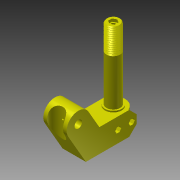
# Autodesk Inventor part: hub bottom
Saved by Autodesk Inventor 2013 (Build 170138000, 138)
## iProperties
Created: 2013-07-14
Part Number: hub bottom
Material: Generic
Document SubType Name: Modeling
Designer: employee
Density: 1 g/cm^3
Author: employee
Autodesk Inventor part; units mm, degrees
ref_plane "YZ Plane" through (0, 0, 0) normal (1, 0, 0) x (0, 1, 0)
ref_plane "XZ Plane" through (0, 0, 0) normal (0, 1, 0) x (-1, 0, 0)
ref_plane "XY Plane" through (0, 0, 0) normal (0, 0, 1) x (1, 0, 0)
sketch "Sketch1" plane through (0, 0, 0) normal (1, 0, 0) x (0, 1, 0)
  circle A0 centre (-50, 14) radius 4.05
  arc A1 (-39.174682, 20.25) -> (-60.825318, 7.75) centre (-50, 14) ccw
  line L0 (0, 0) -> (0, -25)
  line L1 (0, -25) -> (-41.917096, -25)
  line L2 (-41.917096, -25) -> (-60.825318, 7.75)
  line L3 (0, 0) -> (-27.48334, 0)
  line L4 (-27.48334, 0) -> (-39.174682, 20.25)
  dimension "d0" = 8.1
  dimension "d2" = 50
  dimension "d3" = 14
  dimension "d4" = 25
  dimension "d6" = 25
  dimension "d40" = 120
  constraints: 10 end point, 2 centre point, 2 parallel, 2 point on circle, 2 tangent, 1 coincident, 1 perpendicular, 1 vertical
  measures "d0" diameter of A0
  measures "d2" horizontal distance of L0.start A0.centre
  measures "d3" vertical distance of A0.centre L0.start
  measures "d4" diameter of A1
  measures "d6" distance of L0.start L0.end
  measures "d40" angle of L2 L1
extrude "Extrusion1" add sketch "Sketch1" along normal mid plane 25
sketch "Sketch2" plane through (-12.5, -27.48334, 0) normal (0, 0, 1) x (1, 0, 0)
  circle A0 centre (12.5, 27.48334) radius 12.5
  constraints: 1 centre point, 1 coincident
extrude "Extrusion2" add sketch "Sketch2" against normal up to surface (25 mm away)
sketch "Sketch13" plane through (12.5, 0, 0) normal (1, 0, 0) x (0, 0, -1)
  line L0 (0, 0) -> (0, -27.48334)
  line L1 (25, 0) -> (0, 0)
  line L2 (25, 0) -> (25, 0)
  line L3 (0, 0) -> (25, 0)
  line L4 (0, 0) -> (0, 0)
  line L5 (0, 12.5) -> (25, 12.5)
  line L6 (0, 0) -> (0, 12.5)
  line L7 (25, 12.5) -> (25, 0)
  line L8 (0, 4.5) -> (8, 12.5)
  line L9 (17, 12.5) -> (25, 4.5)
  line L10 (0, 0) -> (0, 4.5)
  line L11 (0, 0) -> (25, 0)
  line L12 (25, 0) -> (25, 4.5)
  line L13 (17, 12.5) -> (8, 12.5)
  dimension "d60" = 45
  dimension "d61" = 9
  constraints: 12 end point, 4 perpendicular, 4 point on line, 1 collinear, 1 parallel
  measures "d60" angle of L5 L8
  measures "d61" distance of L9.start L8.end
extrude "Extrusion13" add sketch "Sketch13" against normal up to surface (25 mm away) contours L1 L6 L8 L5 L9 L7
sketch "Sketch12" plane through (12.5, -41.917096, -25) normal (0, 0, -1) x (-1, 0, 0)
  arc A0 (25, 41.917096) -> (0, 41.917096) centre (12.5, 41.917096) ccw
  circle A1 centre (12.5, 41.917096) radius 8.1
  dimension "d56" = 16.2
  constraints: 1 centre point, 1 coincident
  measures "d56" diameter of A1
extrude "Extrusion12" cut sketch "Sketch12" against normal blind 19
sketch "Sketch14" plane through (-12.5, 0, 0) normal (-1, 0, 0) x (0, 0, 1)
  line L0 (-8, 12.5) -> (-17, 12.5) projected
  line L1 (-6, -8.1) -> (-6, 8.1) projected
  line L2 (-25, -8.1) -> (-25, 8.1) projected
  line L3 (-25, 8.1) -> (-6, 8.1) projected
  line L4 (-25, -8.1) -> (-6, -8.1) projected
  line L5 (-12.5, 7.25) -> (-12.5, -7.25)
  circle A0 centre (-12.5, 7.25) radius 1.55
  circle A1 centre (-12.5, -7.25) radius 1.55
  point P0 (0, 0)
  point P1 (-6, -0.010608)
  point P2 (-6, 0)
  point P3 (-12.5, 0)
  point P4 (-12.5, 12.5)
  dimension "d65" = 3.1
  dimension "d67" = 14.5
  constraints: 3 midpoint, 2 centre point, 2 coincident, 2 end point, 2 vertical alignment, 1 equal radius, 1 horizontal alignment, 1 perpendicular
  measures "d65" diameter of A1
  measures "d67" distance of L5.start L5.end
extrude "Extrusion14" cut sketch "Sketch14" against normal through all contours A1 L4 | L4 A1 | A0 L3 | L3 A0
sketch "Sketch15" plane through (-12.5, 0, 0) normal (-1, 0, 0) x (0, 0, 1)
  circle A0 centre (-12.5, -7.25) radius 1.55 projected
  circle A1 centre (-12.5, 7.25) radius 1.55 projected
  circle A2 centre (-12.5, 7.25) radius 3.25
  circle A3 centre (-12.5, -7.25) radius 3.25
  point P0 (0, 0)
  dimension "d70" = 6.5
  constraints: 2 centre point, 2 coincident, 1 equal radius
  measures "d70" diameter of A3
extrude "Extrusion15" cut sketch "Sketch15" against normal blind 4
sketch "Sketch16" plane through (12.5, 0, 0) normal (1, 0, 0) x (0, 0, -1)
  circle A0 centre (12.5, -7.25) radius 1.55
  circle A1 centre (12.5, 7.25) radius 1.55
  line L0 (12.5, -10.483162) -> (9.7, -8.866581)
  line L1 (9.7, -8.866581) -> (9.7, -5.633419)
  line L2 (9.7, -5.633419) -> (12.5, -4.016838)
  line L3 (12.5, -4.016838) -> (15.3, -5.633419)
  line L4 (15.3, -5.633419) -> (15.3, -8.866581)
  line L5 (15.3, -8.866581) -> (12.5, -10.483162)
  line L6 (12.5, 4.016838) -> (9.7, 5.633419)
  line L7 (9.7, 5.633419) -> (9.7, 8.866581)
  line L8 (9.7, 8.866581) -> (12.5, 10.483162)
  line L9 (12.5, 10.483162) -> (15.3, 8.866581)
  line L10 (15.3, 8.866581) -> (15.3, 5.633419)
  line L11 (15.3, 5.633419) -> (12.5, 4.016838)
  point P0 (0, 0)
  dimension "d74" = 5.6
  constraints: 24 end point, 2 coincident, 2 vertical, 1 collinear, 26 other
  measures "d74" distance between parallel lines of L4 L1
extrude "Extrusion16" cut sketch "Sketch16" against normal blind 4
sketch "Sketch17" plane through (-12.5, -27.48334, 0) normal (0, 0, 1) x (1, 0, 0)
  arc A0 (24.161904, 31.98334) -> (0.838096, 31.98334) centre (12.5, 27.48334) ccw
  circle A1 centre (12.5, 27.48334) radius 9
  point P0 (23.286001, 33.800949)
  point P1 (1.713999, 33.800949)
  dimension "d77" = 18
  constraints: 1 centre point, 1 coincident
  measures "d77" diameter of A1
extrude "Extrusion17" add sketch "Sketch17" along normal blind 1.5
sketch "Sketch18" plane through (0, 0, 1.5) normal (0, 0, 1) x (1, 0, 0)
  circle A0 centre (0, 0) radius 9 projected
  circle A1 centre (0, 0) radius 7.35
  dimension "d82" = 14.7
  constraints: 1 centre point, 1 coincident
  measures "d82" diameter of A1
extrude "Extrusion18" add sketch "Sketch18" along normal blind 76.5 contours A1
sketch "Sketch19" plane through (0, 0, 0) normal (1, 0, 0) x (0, 1, 0)
  line L0 (12.5, -17) -> (12.5, -25)
  line L1 (12.5, -25) -> (8.1, -25)
  line L2 (8.1, -25) -> (8.1, -13.796148)
  arc A0 (8.1, -13.796148) -> (8.1, -11.203852) centre (7.25, -12.5) ccw
  line L3 (8.1, -11.203852) -> (8.1, -6)
  line L4 (8.1, -6) -> (-8.1, -6)
  line L5 (-8.1, -6) -> (-8.1, -11.203852)
  arc A1 (-8.1, -11.203852) -> (-8.1, -13.796148) centre (-7.25, -12.5) ccw
  line L6 (-8.1, -13.796148) -> (-8.1, -25)
  line L7 (-8.1, -25) -> (-41.917096, -25)
  line L8 (-41.917096, -25) -> (-60.825318, 7.75)
  arc A2 (-39.174682, 20.25) -> (-60.825318, 7.75) centre (-50, 14) ccw
  line L9 (-39.174682, 20.25) -> (-27.48334, 0)
  line L10 (-27.48334, 0) -> (-9, 0)
  line L11 (-9, 0) -> (-9, 1.5)
  line L12 (-9, 1.5) -> (-7.35, 1.5)
  line L13 (-7.35, 1.5) -> (-7.35, 78)
  line L14 (-7.35, 78) -> (7.35, 78)
  line L15 (7.35, 78) -> (7.35, 1.5)
  line L16 (7.35, 1.5) -> (9, 1.5)
  line L17 (9, 1.5) -> (9, 0)
  line L18 (9, 0) -> (12.5, 0)
  line L19 (12.5, 0) -> (12.5, -8)
  line L20 (12.5, -8) -> (12.5, -17)
  circle A3 centre (-50, 14) radius 4.05
  line L21 (7.35, 78) -> (7.35, 80)
  line L22 (7.35, 80) -> (6.35, 79)
  line L23 (6.35, 79) -> (7.35, 78)
  line L24 (0, 78) -> (0, 72.188815)
  point P0 (0, 0)
  dimension "d87" = 2
  constraints: 8 end point, 2 parallel, 2 perpendicular, 1 midpoint
  measures "d87" distance of L14.end L21.end
coil "Coil1" sketch "Sketch19" operation cut axis through (0, 0, 78) along (0, 0, -1) pitch 2.001 turns 30 hand right contours L23 L22 L21
sketch "Sketch20" plane through (0, 0, 1.5) normal (0, 0, 1) x (1, 0, 0)
  circle A0 centre (0, 0) radius 7.35 projected
extrude "Extrusion19" add sketch "Sketch20" along normal blind 49.5
sketch "Sketch21" plane through (0, 0, 51) normal (0, 0, 1) x (1, 0, 0)
  arc A0 (0.334532, -7.342383) -> (0.311475, -7.343397) centre (0, 0) ccw
  circle A1 centre (0, 0) radius 7.35
  constraints: 1 centre point, 1 coincident, 1 concentric
extrude "Extrusion20" add sketch "Sketch21" along normal blind 5 draft -45
sketch "Sketch22" plane through (0, 0, 78) normal (0, 0, 1) x (1, 0, 0)
  arc A0 (0, 7.35) -> (-0.023079, 7.349964) centre (0, 0) ccw
  circle A1 centre (0, 0) radius 6.45
  circle A2 centre (0, 0) radius 20
  dimension "d100" = 40
  constraints: 2 centre point, 2 coincident
  measures "d100" diameter of A2
extrude "Extrusion21" cut sketch "Sketch22" against normal blind 5 draft -45
sketch "Sketch23" plane through (0, 0, 78) normal (0, 0, 1) x (-0.9999988, -0.00157, 0)
  circle A0 centre (0, 0) radius 6.45 projected
  circle A1 centre (0, 0) radius 2.5
  point P0 (0.010127, -6.449992)
  dimension "d104" = 5
  constraints: 1 centre point, 1 coincident, 1 other
  measures "d104" diameter of A1
extrude "Extrusion22" cut sketch "Sketch23" against normal through all contours A1
sketch "Sketch24" plane through (0, 0, -6) normal (0, 0, -1) x (-1, 0, 0)
  circle A0 centre (0, 0) radius 2.5 projected
extrude "Extrusion23" add sketch "Sketch24" against normal blind 0.4
sketch "Sketch25" plane through (-12.5, 0, 0) normal (-1, 0, 0) x (0, 0, 1)
  circle A0 centre (14, -50) radius 4.05
  arc A1 (8.5, -59.526279) -> (19.5, -40.473721) centre (14, -50) ccw
  line L0 (7.4, -53.810512) -> (7.4, -46.189488)
  line L1 (7.4, -46.189488) -> (14, -42.378976)
  line L2 (14, -42.378976) -> (20.6, -46.189488)
  line L3 (20.6, -46.189488) -> (20.6, -53.810512)
  line L4 (20.6, -53.810512) -> (14, -57.621024)
  line L5 (14, -57.621024) -> (7.4, -53.810512)
  point P0 (0, 0)
  dimension "d117" = 13.2
  constraints: 12 end point, 1 coincident, 1 vertical, 13 other
  measures "d117" distance between parallel lines of L3 L0
extrude "Extrusion24" cut sketch "Sketch25" against normal blind 5.5
sketch "Sketch26" plane through (12.5, -41.917096, -25) normal (0, 0, -1) x (-1, 0, 0)
  line L0 (25, -20.582904) -> (0, -20.582904)
  circle A0 centre (12.5, -20.582904) radius 8.5
  dimension "d120" = 17
  constraints: 1 centre point, 1 midpoint
  measures "d120" diameter of A0
extrude "Extrusion25" cut sketch "Sketch26" against normal through all
sketch "Sketch27" plane through (0, 0, 78) normal (0, 0, 1) x (1, 0, 0)
  circle A0 centre (0, 0) radius 2.5
  arc A1 (2.001825, -6.131492) -> (-1.982563, -6.137748) centre (0, 0) ccw
  line L0 (0, 4.156922) -> (3.6, 2.078461)
  line L1 (3.6, 2.078461) -> (3.6, -2.078461)
  line L2 (3.6, -2.078461) -> (0, -4.156922)
  line L3 (0, -4.156922) -> (-3.6, -2.078461)
  line L4 (-3.6, -2.078461) -> (-3.6, 2.078461)
  line L5 (-3.6, 2.078461) -> (0, 4.156922)
  dimension "d125" = 7.2
  constraints: 12 end point, 1 coincident, 1 vertical, 13 other
  measures "d125" distance between parallel lines of L1 L4
extrude "Extrusion26" cut sketch "Sketch27" against normal blind 3
body "Solid1"
